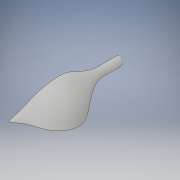
# Autodesk Inventor part: Lotus_Petal
Saved by Autodesk Inventor 2019 (Build 230136000, 136)
## iProperties
Created: 2019-11-09
Part Number: Lotus_Petal
Material: Generic
Document SubType Name: Modeling
Designer: Jorian Brusind
Density: 1 g/cm^3
Appearance: Default
Author: Jorian Brusind
Autodesk Inventor part; units mm, degrees
ref_plane "YZ Plane" through (0, 0, 0) normal (1, 0, 0) x (0, 1, 0)
ref_plane "XZ Plane" through (0, 0, 0) normal (0, 1, 0) x (-1, 0, 0)
ref_plane "XY Plane" through (0, 0, 0) normal (0, 0, 1) x (1, 0, 0)
sketch "Sketch1" plane through (0, 0, 0) normal (0, 1, 0) x (-1, 0, 0)
  line L0 (0, 0) -> (0, -100)
  line L1 (-30, 0) -> (-10, 0) construction
  line L2 (177.9613, -119.7528) -> (-149.4388, -126.0094) construction
  line L3 (-149.4388, -126.0094) -> (-153.9249, 108.7365) construction
  line L4 (-153.9249, 108.7365) -> (173.4753, 114.9931) construction
  line L5 (173.4753, 114.9931) -> (177.9613, -119.7528) construction
  spline S0 degree 4 poles (0, 0) (-2.5173, 0.2484) (-10.3838, -9.1911) (-21.2727, -7.2678) (-35.5405, -18.3704) (-41.7317, -33.7494) (-25.8113, -50.768) (-2.4697, -82.4968) (-8.5728, -85.7499) (-10.0423, -111.6065) (0, -100) knots 0 0 0 0 0 0.198295 0.292373 0.397831 0.519264 0.640217 0.761452 1 1 1 1 1
  point P0 (-4.5659, -2.3798)
  point P1 (-13.6711, -7.521)
  point P2 (-23.2966, -10.6678)
  point P3 (-33.1071, -17.9794)
  point P4 (-37.7347, -30.659)
  point P5 (-26.0731, -51.3907)
  point P6 (-9.2286, -76.3798)
  point P7 (-7.7478, -88.0414)
  point P8 (-7.2851, -101.8316)
  dimension "d0" = 100
  constraints: 4 end point, 1 horizontal, 1 vertical, 13 other
  measures "d0" distance of L0.start L0.end
revolve "Revolution9" add sketch "Sketch1" angle 60 about axis through (0, 0, 0) along (0, 0, 1)
sketch "Sketch7" plane through (0, 0, -100) normal (-0.8660254, 0.5, 0) x (0, 0, 1)
  line L0 (100, 0) -> (0, 0) projected
  spline S0 degree 4 poles (100, 0) (93.1917, 0.9822) (92.8339, 14.9227) (76.9709, 45.0336) (54.445, 23.5944) (41.4626, 16.6222) (24.4086, 1.0723) (8.5565, 6.3337) (-4.6326, 6.5895) (0, 0) knots 0 0 0 0 0 0.279113 0.407068 0.532007 0.655321 0.771332 1 1 1 1 1
  line L1 (100, 0) -> (0, 0)
  point P0 (94.1772, 5.3133)
  point P1 (85.3872, 23.511)
  point P2 (71.3874, 33.4956)
  point P3 (54.8986, 25.1214)
  point P4 (40.7432, 15.1369)
  point P5 (26.4322, 6.4406)
  point P6 (11.0323, 5.3133)
  point P7 (0, 4.6692)
  constraints: 2 end point, 1 horizontal, 10 other
revolve "Revolution10" cut sketch "Sketch7" angle 60 about axis through (0, 0, 0) along (0, 0, -1)
body "Solid5"
